Autodesk Inventor part; units mm, degrees
(part 3 of 3)
sketch "Sketch3" plane through (0, 0, 0) normal (0, -1, 0) x (1, 0, 0)
  circle A0 centre (-1.1015, 1.1015) radius 0.13 projected
  line L0 (-2.1254, 1.1532) -> (-2.1288, 1.1525) projected
  line L1 (-2.1288, 1.1525) -> (-2.1355, 1.1511) projected
  line L2 (-2.1355, 1.1511) -> (-2.149, 1.1477) projected
  line L3 (-2.149, 1.1477) -> (-2.1625, 1.1437) projected
  line L4 (-2.1625, 1.1437) -> (-2.1761, 1.139) projected
  line L5 (-2.1761, 1.139) -> (-2.1896, 1.1339) projected
  line L6 (-2.1896, 1.1339) -> (-2.2031, 1.1282) projected
  line L7 (-2.2031, 1.1282) -> (-2.2031, 1.0756) projected
  line L8 (-2.2031, 1.0756) -> (-2.1896, 1.0699) projected
  line L9 (-2.1896, 1.0699) -> (-2.1761, 1.0647) projected
  line L10 (-2.1761, 1.0647) -> (-2.1626, 1.0601) projected
  line L11 (-2.1626, 1.0601) -> (-2.1491, 1.0561) projected
  line L12 (-2.1491, 1.0561) -> (-2.1356, 1.0527) projected
  line L13 (-2.1356, 1.0527) -> (-2.1288, 1.0513) projected
  line L14 (-2.1288, 1.0513) -> (-2.1254, 1.0506) projected
  line L15 (-2.1254, 1.0506) -> (-2.1221, 1.05) projected
  line L16 (-2.1221, 1.05) -> (-2.1176, 0.9935) projected
  line L17 (-2.1176, 0.9935) -> (-2.1209, 0.9923) projected
  line L18 (-2.1209, 0.9923) -> (-2.1241, 0.9912) projected
  line L19 (-2.1241, 0.9912) -> (-2.1305, 0.9887) projected
  line L20 (-2.1305, 0.9887) -> (-2.1433, 0.9832) projected
  line L21 (-2.1433, 0.9832) -> (-2.156, 0.9772) projected
  line L22 (-2.156, 0.9772) -> (-2.1687, 0.9705) projected
  line L23 (-2.1687, 0.9705) -> (-2.1812, 0.9633) projected
  line L24 (-2.1812, 0.9633) -> (-2.1936, 0.9556) projected
  line L25 (-2.1936, 0.9556) -> (-2.1854, 0.9035) projected
  line L26 (-2.1854, 0.9035) -> (-2.1712, 0.9) projected
  line L27 (-2.1712, 0.9) -> (-2.1571, 0.897) projected
  line L28 (-2.1571, 0.897) -> (-2.143, 0.8945) projected
  line L29 (-2.143, 0.8945) -> (-2.129, 0.8927) projected
  line L30 (-2.129, 0.8927) -> (-2.1151, 0.8914) projected
  line L31 (-2.1151, 0.8914) -> (-2.1083, 0.8911) projected
  line L32 (-2.1083, 0.8911) -> (-2.1048, 0.891) projected
  line L33 (-2.1048, 0.891) -> (-2.1014, 0.8909) projected
  line L34 (-2.1014, 0.8909) -> (-2.0882, 0.8357) projected
  line L35 (-2.0882, 0.8357) -> (-2.0912, 0.8341) projected
  line L36 (-2.0912, 0.8341) -> (-2.0942, 0.8325) projected
  line L37 (-2.0942, 0.8325) -> (-2.1002, 0.829) projected
  line L38 (-2.1002, 0.829) -> (-2.112, 0.8216) projected
  line L39 (-2.112, 0.8216) -> (-2.1236, 0.8136) projected
  line L40 (-2.1236, 0.8136) -> (-2.135, 0.8051) projected
  line L41 (-2.135, 0.8051) -> (-2.1462, 0.796) projected
  line L42 (-2.1462, 0.796) -> (-2.1573, 0.7864) projected
  line L43 (-2.1573, 0.7864) -> (-2.1411, 0.7364) projected
  line L44 (-2.1411, 0.7364) -> (-2.1265, 0.7351) projected
  line L45 (-2.1265, 0.7351) -> (-2.112, 0.7344) projected
  line L46 (-2.112, 0.7344) -> (-2.0978, 0.7342) projected
  line L47 (-2.0978, 0.7342) -> (-2.0837, 0.7345) projected
  line L48 (-2.0837, 0.7345) -> (-2.0698, 0.7355) projected
  line L49 (-2.0698, 0.7355) -> (-2.0629, 0.7362) projected
  line L50 (-2.0629, 0.7362) -> (-2.0595, 0.7366) projected
  line L51 (-2.0595, 0.7366) -> (-2.0561, 0.7371) projected
  line L52 (-2.0561, 0.7371) -> (-2.0344, 0.6847) projected
  line L53 (-2.0344, 0.6847) -> (-2.0371, 0.6826) projected
  line L54 (-2.0371, 0.6826) -> (-2.0398, 0.6805) projected
  line L55 (-2.0398, 0.6805) -> (-2.0452, 0.6762) projected
  line L56 (-2.0452, 0.6762) -> (-2.0557, 0.667) projected
  line L57 (-2.0557, 0.667) -> (-2.0659, 0.6573) projected
  line L58 (-2.0659, 0.6573) -> (-2.0759, 0.6471) projected
  line L59 (-2.0759, 0.6471) -> (-2.0856, 0.6363) projected
  line L60 (-2.0856, 0.6363) -> (-2.095, 0.6252) projected
  line L61 (-2.095, 0.6252) -> (-2.0711, 0.5783) projected
  line L62 (-2.0711, 0.5783) -> (-2.0565, 0.5794) projected
  line L63 (-2.0565, 0.5794) -> (-2.0421, 0.5809) projected
  line L64 (-2.0421, 0.5809) -> (-2.028, 0.5829) projected
  line L65 (-2.028, 0.5829) -> (-2.0141, 0.5855) projected
  line L66 (-2.0141, 0.5855) -> (-2.0006, 0.5886) projected
  line L67 (-2.0006, 0.5886) -> (-1.9939, 0.5903) projected
  line L68 (-1.9939, 0.5903) -> (-1.9906, 0.5913) projected
  line L69 (-1.9906, 0.5913) -> (-1.9873, 0.5923) projected
  line L70 (-1.9873, 0.5923) -> (-1.9577, 0.5439) projected
  line L71 (-1.9577, 0.5439) -> (-1.9601, 0.5415) projected
  line L72 (-1.9601, 0.5415) -> (-1.9624, 0.5389) projected
  line L73 (-1.9624, 0.5389) -> (-1.967, 0.5338) projected
  line L74 (-1.967, 0.5338) -> (-1.976, 0.5231) projected
  line L75 (-1.976, 0.5231) -> (-1.9845, 0.5119) projected
  line L76 (-1.9845, 0.5119) -> (-1.9928, 0.5003) projected
  line L77 (-1.9928, 0.5003) -> (-2.0006, 0.4882) projected
  line L78 (-2.0006, 0.4882) -> (-2.0082, 0.4756) projected
  line L79 (-2.0082, 0.4756) -> (-1.9773, 0.4331) projected
  line L80 (-1.9773, 0.4331) -> (-1.9631, 0.4364) projected
  line L81 (-1.9631, 0.4364) -> (-1.9491, 0.4402) projected
  line L82 (-1.9491, 0.4402) -> (-1.9355, 0.4444) projected
  line L83 (-1.9355, 0.4444) -> (-1.9221, 0.4491) projected
  line L84 (-1.9221, 0.4491) -> (-1.9092, 0.4543) projected
  line L85 (-1.9092, 0.4543) -> (-1.9029, 0.4571) projected
  line L86 (-1.9029, 0.4571) -> (-1.8998, 0.4585) projected
  line L87 (-1.8998, 0.4585) -> (-1.8968, 0.46) projected
  line L88 (-1.8968, 0.46) -> (-1.8599, 0.4169) projected
  line L89 (-1.8599, 0.4169) -> (-1.8619, 0.4141) projected
  line L90 (-1.8619, 0.4141) -> (-1.8638, 0.4112) projected
  line L91 (-1.8638, 0.4112) -> (-1.8675, 0.4054) projected
  line L92 (-1.8675, 0.4054) -> (-1.8747, 0.3935) projected
  line L93 (-1.8747, 0.3935) -> (-1.8814, 0.3811) projected
  line L94 (-1.8814, 0.3811) -> (-1.8877, 0.3683) projected
  line L95 (-1.8877, 0.3683) -> (-1.8936, 0.3551) projected
  line L96 (-1.8936, 0.3551) -> (-1.8991, 0.3415) projected
  line L97 (-1.8991, 0.3415) -> (-1.8619, 0.3043) projected
  line L98 (-1.8619, 0.3043) -> (-1.8484, 0.3099) projected
  line L99 (-1.8484, 0.3099) -> (-1.8352, 0.3158) projected
  line L100 (-1.8352, 0.3158) -> (-1.8224, 0.3221) projected
  line L101 (-1.8224, 0.3221) -> (-1.81, 0.3288) projected
  line L102 (-1.81, 0.3288) -> (-1.798, 0.3359) projected
  line L103 (-1.798, 0.3359) -> (-1.7922, 0.3397) projected
  line L104 (-1.7922, 0.3397) -> (-1.7894, 0.3416) projected
  line L105 (-1.7894, 0.3416) -> (-1.7866, 0.3436) projected
  line L106 (-1.7866, 0.3436) -> (-1.7434, 0.3067) projected
  line L107 (-1.7434, 0.3067) -> (-1.7449, 0.3036) projected
  line L108 (-1.7449, 0.3036) -> (-1.7464, 0.3005) projected
  line L109 (-1.7464, 0.3005) -> (-1.7492, 0.2942) projected
  line L110 (-1.7492, 0.2942) -> (-1.7544, 0.2813) projected
  line L111 (-1.7544, 0.2813) -> (-1.7591, 0.268) projected
  line L112 (-1.7591, 0.268) -> (-1.7633, 0.2544) projected
  line L113 (-1.7633, 0.2544) -> (-1.7671, 0.2404) projected
  line L114 (-1.7671, 0.2404) -> (-1.7704, 0.2261) projected
  line L115 (-1.7704, 0.2261) -> (-1.7278, 0.1952) projected
  line L116 (-1.7278, 0.1952) -> (-1.7153, 0.2028) projected
  line L117 (-1.7153, 0.2028) -> (-1.7032, 0.2107) projected
  line L118 (-1.7032, 0.2107) -> (-1.6915, 0.2189) projected
  line L119 (-1.6915, 0.2189) -> (-1.6803, 0.2275) projected
  line L120 (-1.6803, 0.2275) -> (-1.6696, 0.2364) projected
  line L121 (-1.6696, 0.2364) -> (-1.6645, 0.241) projected
  line L122 (-1.6645, 0.241) -> (-1.662, 0.2434) projected
  line L123 (-1.662, 0.2434) -> (-1.6596, 0.2458) projected
  line L124 (-1.6596, 0.2458) -> (-1.6112, 0.2161) projected
  line L125 (-1.6112, 0.2161) -> (-1.6122, 0.2128) projected
  line L126 (-1.6122, 0.2128) -> (-1.6131, 0.2095) projected
  line L127 (-1.6131, 0.2095) -> (-1.6149, 0.2029) projected
  line L128 (-1.6149, 0.2029) -> (-1.618, 0.1893) projected
  line L129 (-1.618, 0.1893) -> (-1.6206, 0.1754) projected
  line L130 (-1.6206, 0.1754) -> (-1.6226, 0.1613) projected
  line L131 (-1.6226, 0.1613) -> (-1.6241, 0.1469) projected
  line L132 (-1.6241, 0.1469) -> (-1.6252, 0.1323) projected
  line L133 (-1.6252, 0.1323) -> (-1.5783, 0.1084) projected
  line L134 (-1.5783, 0.1084) -> (-1.5671, 0.1179) projected
  line L135 (-1.5671, 0.1179) -> (-1.5564, 0.1276) projected
  line L136 (-1.5564, 0.1276) -> (-1.5462, 0.1375) projected
  line L137 (-1.5462, 0.1375) -> (-1.5364, 0.1477) projected
  line L138 (-1.5364, 0.1477) -> (-1.5273, 0.1582) projected
  line L139 (-1.5273, 0.1582) -> (-1.5229, 0.1636) projected
  line L140 (-1.5229, 0.1636) -> (-1.5208, 0.1663) projected
  line L141 (-1.5208, 0.1663) -> (-1.5188, 0.169) projected
  line L142 (-1.5188, 0.169) -> (-1.4663, 0.1473) projected
  line L143 (-1.4663, 0.1473) -> (-1.4668, 0.1439) projected
  line L144 (-1.4668, 0.1439) -> (-1.4673, 0.1405) projected
  line L145 (-1.4673, 0.1405) -> (-1.468, 0.1337) projected
  line L146 (-1.468, 0.1337) -> (-1.4689, 0.1198) projected
  line L147 (-1.4689, 0.1198) -> (-1.4693, 0.1057) projected
  line L148 (-1.4693, 0.1057) -> (-1.469, 0.0914) projected
  line L149 (-1.469, 0.0914) -> (-1.4683, 0.077) projected
  line L150 (-1.4683, 0.077) -> (-1.4671, 0.0624) projected
  line L151 (-1.4671, 0.0624) -> (-1.4171, 0.0461) projected
  line L152 (-1.4171, 0.0461) -> (-1.4075, 0.0572) projected
  line L153 (-1.4075, 0.0572) -> (-1.3984, 0.0684) projected
  line L154 (-1.3984, 0.0684) -> (-1.3898, 0.0799) projected
  line L155 (-1.3898, 0.0799) -> (-1.3818, 0.0915) projected
  line L156 (-1.3818, 0.0915) -> (-1.3744, 0.1033) projected
  line L157 (-1.3744, 0.1033) -> (-1.371, 0.1092) projected
  line L158 (-1.371, 0.1092) -> (-1.3693, 0.1123) projected
  line L159 (-1.3693, 0.1123) -> (-1.3677, 0.1153) projected
  line L160 (-1.3677, 0.1153) -> (-1.3126, 0.102) projected
  line L161 (-1.3126, 0.102) -> (-1.3125, 0.0986) projected
  line L162 (-1.3125, 0.0986) -> (-1.3124, 0.0952) projected
  line L163 (-1.3124, 0.0952) -> (-1.312, 0.0883) projected
  line L164 (-1.312, 0.0883) -> (-1.3108, 0.0744) projected
  line L165 (-1.3108, 0.0744) -> (-1.3089, 0.0604) projected
  line L166 (-1.3089, 0.0604) -> (-1.3065, 0.0464) projected
  line L167 (-1.3065, 0.0464) -> (-1.3035, 0.0322) projected
  line L168 (-1.3035, 0.0322) -> (-1.3, 0.018) projected
  line L169 (-1.3, 0.018) -> (-1.248, 0.0098) projected
  line L170 (-1.248, 0.0098) -> (-1.2403, 0.0222) projected
  line L171 (-1.2403, 0.0222) -> (-1.2331, 0.0348) projected
  line L172 (-1.2331, 0.0348) -> (-1.2264, 0.0474) projected
  line L173 (-1.2264, 0.0474) -> (-1.2203, 0.0601) projected
  line L174 (-1.2203, 0.0601) -> (-1.2149, 0.0729) projected
  line L175 (-1.2149, 0.0729) -> (-1.2124, 0.0793) projected
  line L176 (-1.2124, 0.0793) -> (-1.2112, 0.0826) projected
  line L177 (-1.2112, 0.0826) -> (-1.2101, 0.0858) projected
  line L178 (-1.2101, 0.0858) -> (-1.1536, 0.0814) projected
  line L179 (-1.1536, 0.0814) -> (-1.153, 0.078) projected
  line L180 (-1.153, 0.078) -> (-1.1523, 0.0746) projected
  line L181 (-1.1523, 0.0746) -> (-1.1509, 0.0679) projected
  line L182 (-1.1509, 0.0679) -> (-1.1475, 0.0544) projected
  line L183 (-1.1475, 0.0544) -> (-1.1435, 0.0409) projected
  line L184 (-1.1435, 0.0409) -> (-1.1389, 0.0273) projected
  line L185 (-1.1389, 0.0273) -> (-1.1337, 0.0138) projected
  line L186 (-1.1337, 0.0138) -> (-1.128, 0.0003) projected
  line L187 (-1.128, 0.0003) -> (-1.0754, 0.0003) projected
  line L188 (-1.0754, 0.0003) -> (-1.0697, 0.0138) projected
  line L189 (-1.0697, 0.0138) -> (-1.0646, 0.0273) projected
  line L190 (-1.0646, 0.0273) -> (-1.06, 0.0409) projected
  line L191 (-1.06, 0.0409) -> (-1.0559, 0.0544) projected
  line L192 (-1.0559, 0.0544) -> (-1.0525, 0.0679) projected
  line L193 (-1.0525, 0.0679) -> (-1.0511, 0.0746) projected
  line L194 (-1.0511, 0.0746) -> (-1.0505, 0.078) projected
  line L195 (-1.0505, 0.078) -> (-1.0499, 0.0814) projected
  line L196 (-1.0499, 0.0814) -> (-0.9933, 0.0858) projected
  line L197 (-0.9933, 0.0858) -> (-0.9922, 0.0826) projected
  line L198 (-0.9922, 0.0826) -> (-0.991, 0.0793) projected
  line L199 (-0.991, 0.0793) -> (-0.9886, 0.0729) projected
  line L200 (-0.9886, 0.0729) -> (-0.9831, 0.0601) projected
  line L201 (-0.9831, 0.0601) -> (-0.977, 0.0474) projected
  line L202 (-0.977, 0.0474) -> (-0.9703, 0.0348) projected
  line L203 (-0.9703, 0.0348) -> (-0.9631, 0.0222) projected
  line L204 (-0.9631, 0.0222) -> (-0.9554, 0.0098) projected
  line L205 (-0.9554, 0.0098) -> (-0.9034, 0.018) projected
  line L206 (-0.9034, 0.018) -> (-0.9, 0.0322) projected
  line L207 (-0.9, 0.0322) -> (-0.897, 0.0464) projected
  line L208 (-0.897, 0.0464) -> (-0.8945, 0.0604) projected
  line L209 (-0.8945, 0.0604) -> (-0.8927, 0.0744) projected
  line L210 (-0.8927, 0.0744) -> (-0.8914, 0.0883) projected
  line L211 (-0.8914, 0.0883) -> (-0.8911, 0.0952) projected
  line L212 (-0.8911, 0.0952) -> (-0.891, 0.0986) projected
  line L213 (-0.891, 0.0986) -> (-0.8909, 0.102) projected
  line L214 (-0.8909, 0.102) -> (-0.8357, 0.1153) projected
  line L215 (-0.8357, 0.1153) -> (-0.8341, 0.1123) projected
  line L216 (-0.8341, 0.1123) -> (-0.8325, 0.1093) projected
  line L217 (-0.8325, 0.1093) -> (-0.829, 0.1033) projected
  line L218 (-0.829, 0.1033) -> (-0.8216, 0.0915) projected
  line L219 (-0.8216, 0.0915) -> (-0.8136, 0.0799) projected
  line L220 (-0.8136, 0.0799) -> (-0.805, 0.0685) projected
  line L221 (-0.805, 0.0685) -> (-0.796, 0.0572) projected
  line L222 (-0.796, 0.0572) -> (-0.7864, 0.0461) projected
  line L223 (-0.7864, 0.0461) -> (-0.7364, 0.0624) projected
  line L224 (-0.7364, 0.0624) -> (-0.7351, 0.077) projected
  line L225 (-0.7351, 0.077) -> (-0.7344, 0.0914) projected
  line L226 (-0.7344, 0.0914) -> (-0.7342, 0.1057) projected
  line L227 (-0.7342, 0.1057) -> (-0.7345, 0.1198) projected
  line L228 (-0.7345, 0.1198) -> (-0.7355, 0.1337) projected
  line L229 (-0.7355, 0.1337) -> (-0.7362, 0.1405) projected
  line L230 (-0.7362, 0.1405) -> (-0.7366, 0.1439) projected
  line L231 (-0.7366, 0.1439) -> (-0.7371, 0.1473) projected
  line L232 (-0.7371, 0.1473) -> (-0.6847, 0.169) projected
  line L233 (-0.6847, 0.169) -> (-0.6826, 0.1663) projected
  line L234 (-0.6826, 0.1663) -> (-0.6805, 0.1636) projected
  line L235 (-0.6805, 0.1636) -> (-0.6762, 0.1582) projected
  line L236 (-0.6762, 0.1582) -> (-0.667, 0.1477) projected
  line L237 (-0.667, 0.1477) -> (-0.6573, 0.1375) projected
  line L238 (-0.6573, 0.1375) -> (-0.647, 0.1276) projected
  line L239 (-0.647, 0.1276) -> (-0.6363, 0.1179) projected
  line L240 (-0.6363, 0.1179) -> (-0.6251, 0.1084) projected
  line L241 (-0.6251, 0.1084) -> (-0.5783, 0.1323) projected
  line L242 (-0.5783, 0.1323) -> (-0.5793, 0.1469) projected
  line L243 (-0.5793, 0.1469) -> (-0.5809, 0.1613) projected
  line L244 (-0.5809, 0.1613) -> (-0.5829, 0.1754) projected
  line L245 (-0.5829, 0.1754) -> (-0.5854, 0.1893) projected
  line L246 (-0.5854, 0.1893) -> (-0.5885, 0.2029) projected
  line L247 (-0.5885, 0.2029) -> (-0.5903, 0.2095) projected
  line L248 (-0.5903, 0.2095) -> (-0.5913, 0.2128) projected
  line L249 (-0.5913, 0.2128) -> (-0.5923, 0.2161) projected
  line L250 (-0.5923, 0.2161) -> (-0.5439, 0.2457) projected
  line L251 (-0.5439, 0.2457) -> (-0.5414, 0.2434) projected
  line L252 (-0.5414, 0.2434) -> (-0.5389, 0.241) projected
  line L253 (-0.5389, 0.241) -> (-0.5338, 0.2364) projected
  line L254 (-0.5338, 0.2364) -> (-0.5231, 0.2275) projected
  line L255 (-0.5231, 0.2275) -> (-0.5119, 0.2189) projected
  line L256 (-0.5119, 0.2189) -> (-0.5002, 0.2107) projected
  line L257 (-0.5002, 0.2107) -> (-0.4881, 0.2028) projected
  line L258 (-0.4881, 0.2028) -> (-0.4756, 0.1952) projected
  line L259 (-0.4756, 0.1952) -> (-0.4331, 0.2261) projected
  line L260 (-0.4331, 0.2261) -> (-0.4364, 0.2404) projected
  line L261 (-0.4364, 0.2404) -> (-0.4402, 0.2543) projected
  line L262 (-0.4402, 0.2543) -> (-0.4444, 0.268) projected
  line L263 (-0.4444, 0.268) -> (-0.449, 0.2813) projected
  line L264 (-0.449, 0.2813) -> (-0.4542, 0.2942) projected
  line L265 (-0.4542, 0.2942) -> (-0.457, 0.3005) projected
  line L266 (-0.457, 0.3005) -> (-0.4585, 0.3036) projected
  line L267 (-0.4585, 0.3036) -> (-0.46, 0.3067) projected
  line L268 (-0.46, 0.3067) -> (-0.4168, 0.3435) projected
  line L269 (-0.4168, 0.3435) -> (-0.414, 0.3416) projected
  line L270 (-0.414, 0.3416) -> (-0.4112, 0.3396) projected
  line L271 (-0.4112, 0.3396) -> (-0.4054, 0.3359) projected
  line L272 (-0.4054, 0.3359) -> (-0.3935, 0.3287) projected
  line L273 (-0.3935, 0.3287) -> (-0.3811, 0.322) projected
  line L274 (-0.3811, 0.322) -> (-0.3683, 0.3157) projected
  line L275 (-0.3683, 0.3157) -> (-0.3551, 0.3098) projected
  line L276 (-0.3551, 0.3098) -> (-0.3415, 0.3043) projected
  line L277 (-0.3415, 0.3043) -> (-0.3043, 0.3415) projected
  line L278 (-0.3043, 0.3415) -> (-0.3098, 0.3551) projected
  line L279 (-0.3098, 0.3551) -> (-0.3157, 0.3683) projected
  line L280 (-0.3157, 0.3683) -> (-0.322, 0.3811) projected
  line L281 (-0.322, 0.3811) -> (-0.3287, 0.3935) projected
  line L282 (-0.3287, 0.3935) -> (-0.3359, 0.4054) projected
  line L283 (-0.3359, 0.4054) -> (-0.3396, 0.4112) projected
  line L284 (-0.3396, 0.4112) -> (-0.3416, 0.4141) projected
  line L285 (-0.3416, 0.4141) -> (-0.3435, 0.4169) projected
  line L286 (-0.3435, 0.4169) -> (-0.3067, 0.46) projected
  line L287 (-0.3067, 0.46) -> (-0.3036, 0.4585) projected
  line L288 (-0.3036, 0.4585) -> (-0.3005, 0.457) projected
  line L289 (-0.3005, 0.457) -> (-0.2942, 0.4542) projected
  line L290 (-0.2942, 0.4542) -> (-0.2813, 0.449) projected
  line L291 (-0.2813, 0.449) -> (-0.268, 0.4444) projected
  line L292 (-0.268, 0.4444) -> (-0.2543, 0.4402) projected
  line L293 (-0.2543, 0.4402) -> (-0.2404, 0.4364) projected
  line L294 (-0.2404, 0.4364) -> (-0.2261, 0.4331) projected
  line L295 (-0.2261, 0.4331) -> (-0.1952, 0.4756) projected
  line L296 (-0.1952, 0.4756) -> (-0.2028, 0.4881) projected
  line L297 (-0.2028, 0.4881) -> (-0.2107, 0.5002) projected
  line L298 (-0.2107, 0.5002) -> (-0.2189, 0.5119) projected
  line L299 (-0.2189, 0.5119) -> (-0.2275, 0.5231) projected
  line L300 (-0.2275, 0.5231) -> (-0.2364, 0.5338) projected
  line L301 (-0.2364, 0.5338) -> (-0.241, 0.5389) projected
  line L302 (-0.241, 0.5389) -> (-0.2434, 0.5414) projected
  line L303 (-0.2434, 0.5414) -> (-0.2457, 0.5439) projected
  line L304 (-0.2457, 0.5439) -> (-0.2161, 0.5923) projected
  line L305 (-0.2161, 0.5923) -> (-0.2128, 0.5913) projected
  line L306 (-0.2128, 0.5913) -> (-0.2095, 0.5903) projected
  line L307 (-0.2095, 0.5903) -> (-0.2029, 0.5885) projected
  line L308 (-0.2029, 0.5885) -> (-0.1893, 0.5854) projected
  line L309 (-0.1893, 0.5854) -> (-0.1754, 0.5829) projected
  line L310 (-0.1754, 0.5829) -> (-0.1613, 0.5809) projected
  line L311 (-0.1613, 0.5809) -> (-0.1469, 0.5793) projected
  line L312 (-0.1469, 0.5793) -> (-0.1323, 0.5782) projected
  line L313 (-0.1323, 0.5782) -> (-0.1084, 0.6251) projected
  line L314 (-0.1084, 0.6251) -> (-0.1179, 0.6363) projected
  line L315 (-0.1179, 0.6363) -> (-0.1276, 0.647) projected
  line L316 (-0.1276, 0.647) -> (-0.1375, 0.6573) projected
  line L317 (-0.1375, 0.6573) -> (-0.1477, 0.667) projected
  line L318 (-0.1477, 0.667) -> (-0.1582, 0.6762) projected
  line L319 (-0.1582, 0.6762) -> (-0.1636, 0.6805) projected
  line L320 (-0.1636, 0.6805) -> (-0.1663, 0.6826) projected
  line L321 (-0.1663, 0.6826) -> (-0.169, 0.6847) projected
  line L322 (-0.169, 0.6847) -> (-0.1473, 0.7371) projected
  line L323 (-0.1473, 0.7371) -> (-0.1439, 0.7366) projected
  line L324 (-0.1439, 0.7366) -> (-0.1405, 0.7362) projected
  line L325 (-0.1405, 0.7362) -> (-0.1336, 0.7355) projected
  line L326 (-0.1336, 0.7355) -> (-0.1197, 0.7345) projected
  line L327 (-0.1197, 0.7345) -> (-0.1056, 0.7342) projected
  line L328 (-0.1056, 0.7342) -> (-0.0914, 0.7344) projected
  line L329 (-0.0914, 0.7344) -> (-0.0769, 0.7351) projected
  line L330 (-0.0769, 0.7351) -> (-0.0624, 0.7363) projected
  line L331 (-0.0624, 0.7363) -> (-0.0461, 0.7864) projected
  line L332 (-0.0461, 0.7864) -> (-0.0572, 0.7959) projected
  line L333 (-0.0572, 0.7959) -> (-0.0684, 0.805) projected
  line L334 (-0.0684, 0.805) -> (-0.0799, 0.8136) projected
  line L335 (-0.0799, 0.8136) -> (-0.0915, 0.8216) projected
  line L336 (-0.0915, 0.8216) -> (-0.1033, 0.829) projected
  line L337 (-0.1033, 0.829) -> (-0.1092, 0.8324) projected
  line L338 (-0.1092, 0.8324) -> (-0.1122, 0.8341) projected
  line L339 (-0.1122, 0.8341) -> (-0.1153, 0.8357) projected
  line L340 (-0.1153, 0.8357) -> (-0.102, 0.8909) projected
  line L341 (-0.102, 0.8909) -> (-0.0986, 0.8909) projected
  line L342 (-0.0986, 0.8909) -> (-0.0952, 0.891) projected
  line L343 (-0.0952, 0.891) -> (-0.0883, 0.8914) projected
  line L344 (-0.0883, 0.8914) -> (-0.0744, 0.8926) projected
  line L345 (-0.0744, 0.8926) -> (-0.0604, 0.8945) projected
  line L346 (-0.0604, 0.8945) -> (-0.0464, 0.897) projected
  line L347 (-0.0464, 0.897) -> (-0.0322, 0.8999) projected
  line L348 (-0.0322, 0.8999) -> (-0.018, 0.9034) projected
  line L349 (-0.018, 0.9034) -> (-0.0098, 0.9554) projected
  line L350 (-0.0098, 0.9554) -> (-0.0222, 0.9631) projected
  line L351 (-0.0222, 0.9631) -> (-0.0347, 0.9703) projected
  line L352 (-0.0347, 0.9703) -> (-0.0474, 0.977) projected
  line L353 (-0.0474, 0.977) -> (-0.0601, 0.9831) projected
  line L354 (-0.0601, 0.9831) -> (-0.0729, 0.9885) projected
  line L355 (-0.0729, 0.9885) -> (-0.0793, 0.991) projected
  line L356 (-0.0793, 0.991) -> (-0.0825, 0.9922) projected
  line L357 (-0.0825, 0.9922) -> (-0.0858, 0.9933) projected
  line L358 (-0.0858, 0.9933) -> (-0.0813, 1.0499) projected
  line L359 (-0.0813, 1.0499) -> (-0.078, 1.0505) projected
  line L360 (-0.078, 1.0505) -> (-0.0746, 1.0511) projected
  line L361 (-0.0746, 1.0511) -> (-0.0678, 1.0525) projected
  line L362 (-0.0678, 1.0525) -> (-0.0543, 1.0559) projected
  line L363 (-0.0543, 1.0559) -> (-0.0408, 1.06) projected
  line L364 (-0.0408, 1.06) -> (-0.0273, 1.0646) projected
  line L365 (-0.0273, 1.0646) -> (-0.0138, 1.0697) projected
  line L366 (-0.0138, 1.0697) -> (-0.0003, 1.0754) projected
  line L367 (-0.0003, 1.0754) -> (-0.0003, 1.128) projected
  line L368 (-0.0003, 1.128) -> (-0.0138, 1.1337) projected
  line L369 (-0.0138, 1.1337) -> (-0.0273, 1.1388) projected
  line L370 (-0.0273, 1.1388) -> (-0.0408, 1.1435) projected
  line L371 (-0.0408, 1.1435) -> (-0.0543, 1.1475) projected
  line L372 (-0.0543, 1.1475) -> (-0.0678, 1.1509) projected
  line L373 (-0.0678, 1.1509) -> (-0.0746, 1.1523) projected
  line L374 (-0.0746, 1.1523) -> (-0.078, 1.153) projected
  line L375 (-0.078, 1.153) -> (-0.0813, 1.1536) projected
  line L376 (-0.0813, 1.1536) -> (-0.0858, 1.2101) projected
  line L377 (-0.0858, 1.2101) -> (-0.0825, 1.2112) projected
  line L378 (-0.0825, 1.2112) -> (-0.0793, 1.2124) projected
  line L379 (-0.0793, 1.2124) -> (-0.0729, 1.2149) projected
  line L380 (-0.0729, 1.2149) -> (-0.0601, 1.2203) projected
  line L381 (-0.0601, 1.2203) -> (-0.0474, 1.2264) projected
  line L382 (-0.0474, 1.2264) -> (-0.0347, 1.2331) projected
  line L383 (-0.0347, 1.2331) -> (-0.0222, 1.2403) projected
  line L384 (-0.0222, 1.2403) -> (-0.0098, 1.248) projected
  line L385 (-0.0098, 1.248) -> (-0.018, 1.3) projected
  line L386 (-0.018, 1.3) -> (-0.0322, 1.3035) projected
  line L387 (-0.0322, 1.3035) -> (-0.0464, 1.3065) projected
  line L388 (-0.0464, 1.3065) -> (-0.0604, 1.3089) projected
  line L389 (-0.0604, 1.3089) -> (-0.0744, 1.3108) projected
  line L390 (-0.0744, 1.3108) -> (-0.0883, 1.312) projected
  line L391 (-0.0883, 1.312) -> (-0.0952, 1.3124) projected
  line L392 (-0.0952, 1.3124) -> (-0.0986, 1.3125) projected
  line L393 (-0.0986, 1.3125) -> (-0.102, 1.3125) projected
  line L394 (-0.102, 1.3125) -> (-0.1153, 1.3677) projected
  line L395 (-0.1153, 1.3677) -> (-0.1122, 1.3693) projected
  line L396 (-0.1122, 1.3693) -> (-0.1092, 1.371) projected
  line L397 (-0.1092, 1.371) -> (-0.1033, 1.3744) projected
  line L398 (-0.1033, 1.3744) -> (-0.0915, 1.3818) projected
  line L399 (-0.0915, 1.3818) -> (-0.0799, 1.3898) projected
  line L400 (-0.0799, 1.3898) -> (-0.0684, 1.3984) projected
  line L401 (-0.0684, 1.3984) -> (-0.0572, 1.4075) projected
  line L402 (-0.0572, 1.4075) -> (-0.0461, 1.417) projected
  line L403 (-0.0461, 1.417) -> (-0.0624, 1.4671) projected
  line L404 (-0.0624, 1.4671) -> (-0.0769, 1.4683) projected
  line L405 (-0.0769, 1.4683) -> (-0.0914, 1.469) projected
  line L406 (-0.0914, 1.469) -> (-0.1056, 1.4692) projected
  line L407 (-0.1056, 1.4692) -> (-0.1197, 1.4689) projected
  line L408 (-0.1197, 1.4689) -> (-0.1336, 1.468) projected
  line L409 (-0.1336, 1.468) -> (-0.1405, 1.4672) projected
  line L410 (-0.1405, 1.4672) -> (-0.1439, 1.4668) projected
  line L411 (-0.1439, 1.4668) -> (-0.1473, 1.4663) projected
  line L412 (-0.1473, 1.4663) -> (-0.169, 1.5188) projected
  line L413 (-0.169, 1.5188) -> (-0.1663, 1.5208) projected
  line L414 (-0.1663, 1.5208) -> (-0.1636, 1.5229) projected
  line L415 (-0.1636, 1.5229) -> (-0.1582, 1.5273) projected
  line L416 (-0.1582, 1.5273) -> (-0.1477, 1.5364) projected
  line L417 (-0.1477, 1.5364) -> (-0.1375, 1.5461) projected
  line L418 (-0.1375, 1.5461) -> (-0.1275, 1.5564) projected
  line L419 (-0.1275, 1.5564) -> (-0.1179, 1.5671) projected
  line L420 (-0.1179, 1.5671) -> (-0.1084, 1.5783) projected
  line L421 (-0.1084, 1.5783) -> (-0.1323, 1.6252) projected
  line L422 (-0.1323, 1.6252) -> (-0.1469, 1.6241) projected
  line L423 (-0.1469, 1.6241) -> (-0.1613, 1.6226) projected
  line L424 (-0.1613, 1.6226) -> (-0.1754, 1.6205) projected
  line L425 (-0.1754, 1.6205) -> (-0.1893, 1.618) projected
  line L426 (-0.1893, 1.618) -> (-0.2028, 1.6149) projected
  line L427 (-0.2028, 1.6149) -> (-0.2095, 1.6131) projected
  line L428 (-0.2095, 1.6131) -> (-0.2128, 1.6122) projected
  line L429 (-0.2128, 1.6122) -> (-0.2161, 1.6112) projected
  line L430 (-0.2161, 1.6112) -> (-0.2457, 1.6595) projected
  line L431 (-0.2457, 1.6595) -> (-0.2433, 1.662) projected
  line L432 (-0.2433, 1.662) -> (-0.241, 1.6645) projected
  line L433 (-0.241, 1.6645) -> (-0.2364, 1.6696) projected
  line L434 (-0.2364, 1.6696) -> (-0.2274, 1.6803) projected
  line L435 (-0.2274, 1.6803) -> (-0.2189, 1.6915) projected
  line L436 (-0.2189, 1.6915) -> (-0.2106, 1.7032) projected
  line L437 (-0.2106, 1.7032) -> (-0.2028, 1.7153) projected
  line L438 (-0.2028, 1.7153) -> (-0.1952, 1.7278) projected
  line L439 (-0.1952, 1.7278) -> (-0.2261, 1.7704) projected
  line L440 (-0.2261, 1.7704) -> (-0.2403, 1.767) projected
  line L441 (-0.2403, 1.767) -> (-0.2543, 1.7633) projected
  line L442 (-0.2543, 1.7633) -> (-0.268, 1.7591) projected
  line L443 (-0.268, 1.7591) -> (-0.2813, 1.7544) projected
  line L444 (-0.2813, 1.7544) -> (-0.2942, 1.7492) projected
  line L445 (-0.2942, 1.7492) -> (-0.3005, 1.7464) projected
  line L446 (-0.3005, 1.7464) -> (-0.3036, 1.7449) projected
  line L447 (-0.3036, 1.7449) -> (-0.3067, 1.7434) projected
  line L448 (-0.3067, 1.7434) -> (-0.3435, 1.7866) projected
  line L449 (-0.3435, 1.7866) -> (-0.3415, 1.7894) projected
  line L450 (-0.3415, 1.7894) -> (-0.3396, 1.7922) projected
  line L451 (-0.3396, 1.7922) -> (-0.3358, 1.798) projected
  line L452 (-0.3358, 1.798) -> (-0.3287, 1.8099) projected
  line L453 (-0.3287, 1.8099) -> (-0.322, 1.8224) projected
  line L454 (-0.322, 1.8224) -> (-0.3157, 1.8352) projected
  line L455 (-0.3157, 1.8352) -> (-0.3098, 1.8484) projected
  line L456 (-0.3098, 1.8484) -> (-0.3043, 1.8619) projected
  line L457 (-0.3043, 1.8619) -> (-0.3415, 1.8991) projected
  line L458 (-0.3415, 1.8991) -> (-0.355, 1.8936) projected
  line L459 (-0.355, 1.8936) -> (-0.3682, 1.8877) projected
  line L460 (-0.3682, 1.8877) -> (-0.381, 1.8814) projected
  line L461 (-0.381, 1.8814) -> (-0.3934, 1.8747) projected
  line L462 (-0.3934, 1.8747) -> (-0.4054, 1.8676) projected
  line L463 (-0.4054, 1.8676) -> (-0.4112, 1.8638) projected
  line L464 (-0.4112, 1.8638) -> (-0.414, 1.8619) projected
  line L465 (-0.414, 1.8619) -> (-0.4168, 1.8599) projected
  line L466 (-0.4168, 1.8599) -> (-0.46, 1.8968) projected
  line L467 (-0.46, 1.8968) -> (-0.4585, 1.8998) projected
  line L468 (-0.4585, 1.8998) -> (-0.457, 1.9029) projected
  line L469 (-0.457, 1.9029) -> (-0.4542, 1.9092) projected
  line L470 (-0.4542, 1.9092) -> (-0.449, 1.9222) projected
  line L471 (-0.449, 1.9222) -> (-0.4443, 1.9355) projected
  line L472 (-0.4443, 1.9355) -> (-0.4401, 1.9491) projected
  line L473 (-0.4401, 1.9491) -> (-0.4363, 1.9631) projected
  line L474 (-0.4363, 1.9631) -> (-0.433, 1.9773) projected
  line L475 (-0.433, 1.9773) -> (-0.4756, 2.0082) projected
  line L476 (-0.4756, 2.0082) -> (-0.4881, 2.0007) projected
  line L477 (-0.4881, 2.0007) -> (-0.5002, 1.9928) projected
  line L478 (-0.5002, 1.9928) -> (-0.5119, 1.9845) projected
  line L479 (-0.5119, 1.9845) -> (-0.5231, 1.976) projected
  line L480 (-0.5231, 1.976) -> (-0.5338, 1.967) projected
  line L481 (-0.5338, 1.967) -> (-0.5389, 1.9624) projected
  line L482 (-0.5389, 1.9624) -> (-0.5414, 1.9601) projected
  line L483 (-0.5414, 1.9601) -> (-0.5438, 1.9577) projected
  line L484 (-0.5438, 1.9577) -> (-0.5922, 1.9874) projected
  line L485 (-0.5922, 1.9874) -> (-0.5912, 1.9906) projected
  line L486 (-0.5912, 1.9906) -> (-0.5903, 1.9939) projected
  line L487 (-0.5903, 1.9939) -> (-0.5885, 2.0006) projected
  line L488 (-0.5885, 2.0006) -> (-0.5854, 2.0142) projected
  line L489 (-0.5854, 2.0142) -> (-0.5828, 2.028) projected
  line L490 (-0.5828, 2.028) -> (-0.5808, 2.0422) projected
  line L491 (-0.5808, 2.0422) -> (-0.5793, 2.0565) projected
  line L492 (-0.5793, 2.0565) -> (-0.5782, 2.0711) projected
  line L493 (-0.5782, 2.0711) -> (-0.6251, 2.095) projected
  line L494 (-0.6251, 2.095) -> (-0.6363, 2.0856) projected
  line L495 (-0.6363, 2.0856) -> (-0.647, 2.0759) projected
  line L496 (-0.647, 2.0759) -> (-0.6572, 2.0659) projected
  line L497 (-0.6572, 2.0659) -> (-0.667, 2.0557) projected
  line L498 (-0.667, 2.0557) -> (-0.6761, 2.0452) projected
  line L499 (-0.6761, 2.0452) -> (-0.6805, 2.0399) projected
  line L500 (-0.6805, 2.0399) -> (-0.6826, 2.0372) projected
  line L501 (-0.6826, 2.0372) -> (-0.6846, 2.0344) projected
  line L502 (-0.6846, 2.0344) -> (-0.737, 2.0562) projected
  line L503 (-0.737, 2.0562) -> (-0.7366, 2.0595) projected
  line L504 (-0.7366, 2.0595) -> (-0.7361, 2.0629) projected
  line L505 (-0.7361, 2.0629) -> (-0.7354, 2.0698) projected
  line L506 (-0.7354, 2.0698) -> (-0.7345, 2.0837) projected
  line L507 (-0.7345, 2.0837) -> (-0.7341, 2.0978) projected
  line L508 (-0.7341, 2.0978) -> (-0.7343, 2.1121) projected
  line L509 (-0.7343, 2.1121) -> (-0.7351, 2.1265) projected
  line L510 (-0.7351, 2.1265) -> (-0.7363, 2.1411) projected
  line L511 (-0.7363, 2.1411) -> (-0.7863, 2.1573) projected
  line L512 (-0.7863, 2.1573) -> (-0.7959, 2.1463) projected
  line L513 (-0.7959, 2.1463) -> (-0.805, 2.135) projected
  line L514 (-0.805, 2.135) -> (-0.8135, 2.1236) projected
  line L515 (-0.8135, 2.1236) -> (-0.8215, 2.112) projected
  line L516 (-0.8215, 2.112) -> (-0.8289, 2.1002) projected
  line L517 (-0.8289, 2.1002) -> (-0.8324, 2.0942) projected
  line L518 (-0.8324, 2.0942) -> (-0.8341, 2.0912) projected
  line L519 (-0.8341, 2.0912) -> (-0.8357, 2.0882) projected
  line L520 (-0.8357, 2.0882) -> (-0.8908, 2.1014) projected
  line L521 (-0.8908, 2.1014) -> (-0.8909, 2.1049) projected
  line L522 (-0.8909, 2.1049) -> (-0.891, 2.1083) projected
  line L523 (-0.891, 2.1083) -> (-0.8914, 2.1152) projected
  line L524 (-0.8914, 2.1152) -> (-0.8926, 2.129) projected
  line L525 (-0.8926, 2.129) -> (-0.8945, 2.143) projected
  line L526 (-0.8945, 2.143) -> (-0.8969, 2.1571) projected
  line L527 (-0.8969, 2.1571) -> (-0.8999, 2.1712) projected
  line L528 (-0.8999, 2.1712) -> (-0.9034, 2.1855) projected
  line L529 (-0.9034, 2.1855) -> (-0.9553, 2.1937) projected
  line L530 (-0.9553, 2.1937) -> (-0.9631, 2.1812) projected
  line L531 (-0.9631, 2.1812) -> (-0.9703, 2.1687) projected
  line L532 (-0.9703, 2.1687) -> (-0.9769, 2.1561) projected
  line L533 (-0.9769, 2.1561) -> (-0.983, 2.1434) projected
  line L534 (-0.983, 2.1434) -> (-0.9885, 2.1306) projected
  line L535 (-0.9885, 2.1306) -> (-0.991, 2.1241) projected
  line L536 (-0.991, 2.1241) -> (-0.9921, 2.1209) projected
  line L537 (-0.9921, 2.1209) -> (-0.9932, 2.1177) projected
  line L538 (-0.9932, 2.1177) -> (-1.0498, 2.1221) projected
  line L539 (-1.0498, 2.1221) -> (-1.0504, 2.1255) projected
  line L540 (-1.0504, 2.1255) -> (-1.0511, 2.1289) projected
  line L541 (-1.0511, 2.1289) -> (-1.0525, 2.1356) projected
  line L542 (-1.0525, 2.1356) -> (-1.0559, 2.1491) projected
  line L543 (-1.0559, 2.1491) -> (-1.0599, 2.1626) projected
  line L544 (-1.0599, 2.1626) -> (-1.0645, 2.1761) projected
  line L545 (-1.0645, 2.1761) -> (-1.0697, 2.1896) projected
  line L546 (-1.0697, 2.1896) -> (-1.0754, 2.2031) projected
  line L547 (-1.0754, 2.2031) -> (-1.128, 2.2031) projected
  line L548 (-1.128, 2.2031) -> (-1.1336, 2.1896) projected
  line L549 (-1.1336, 2.1896) -> (-1.1388, 2.1761) projected
  line L550 (-1.1388, 2.1761) -> (-1.1434, 2.1626) projected
  line L551 (-1.1434, 2.1626) -> (-1.1474, 2.1491) projected
  line L552 (-1.1474, 2.1491) -> (-1.1508, 2.1356) projected
  line L553 (-1.1508, 2.1356) -> (-1.1523, 2.1289) projected
  line L554 (-1.1523, 2.1289) -> (-1.1529, 2.1255) projected
  line L555 (-1.1529, 2.1255) -> (-1.1535, 2.1221) projected
  line L556 (-1.1535, 2.1221) -> (-1.2101, 2.1177) projected
  line L557 (-1.2101, 2.1177) -> (-1.2112, 2.1209) projected
  line L558 (-1.2112, 2.1209) -> (-1.2124, 2.1241) projected
  line L559 (-1.2124, 2.1241) -> (-1.2148, 2.1306) projected
  line L560 (-1.2148, 2.1306) -> (-1.2203, 2.1434) projected
  line L561 (-1.2203, 2.1434) -> (-1.2264, 2.1561) projected
  line L562 (-1.2264, 2.1561) -> (-1.2331, 2.1687) projected
  line L563 (-1.2331, 2.1687) -> (-1.2403, 2.1812) projected
  line L564 (-1.2403, 2.1812) -> (-1.248, 2.1937) projected
  line L565 (-1.248, 2.1937) -> (-1.2999, 2.1855) projected
  line L566 (-1.2999, 2.1855) -> (-1.3034, 2.1712) projected
  line L567 (-1.3034, 2.1712) -> (-1.3064, 2.1571) projected
  line L568 (-1.3064, 2.1571) -> (-1.3089, 2.143) projected
  line L569 (-1.3089, 2.143) -> (-1.3107, 2.129) projected
  line L570 (-1.3107, 2.129) -> (-1.312, 2.1152) projected
  line L571 (-1.312, 2.1152) -> (-1.3123, 2.1083) projected
  line L572 (-1.3123, 2.1083) -> (-1.3124, 2.1049) projected
  line L573 (-1.3124, 2.1049) -> (-1.3125, 2.1014) projected
  line L574 (-1.3125, 2.1014) -> (-1.3677, 2.0882) projected
  line L575 (-1.3677, 2.0882) -> (-1.3693, 2.0912) projected
  line L576 (-1.3693, 2.0912) -> (-1.3709, 2.0942) projected
  line L577 (-1.3709, 2.0942) -> (-1.3744, 2.1002) projected
  line L578 (-1.3744, 2.1002) -> (-1.3818, 2.112) projected
  line L579 (-1.3818, 2.112) -> (-1.3898, 2.1236) projected
  line L580 (-1.3898, 2.1236) -> (-1.3983, 2.135) projected
  line L581 (-1.3983, 2.135) -> (-1.4074, 2.1463) projected
  line L582 (-1.4074, 2.1463) -> (-1.417, 2.1573) projected
  line L583 (-1.417, 2.1573) -> (-1.467, 2.1411) projected
  line L584 (-1.467, 2.1411) -> (-1.4683, 2.1265) projected
  line L585 (-1.4683, 2.1265) -> (-1.469, 2.1121) projected
  line L586 (-1.469, 2.1121) -> (-1.4692, 2.0978) projected
  line L587 (-1.4692, 2.0978) -> (-1.4689, 2.0837) projected
  line L588 (-1.4689, 2.0837) -> (-1.4679, 2.0698) projected
  line L589 (-1.4679, 2.0698) -> (-1.4672, 2.0629) projected
  line L590 (-1.4672, 2.0629) -> (-1.4668, 2.0595) projected
  line L591 (-1.4668, 2.0595) -> (-1.4663, 2.0562) projected
  line L592 (-1.4663, 2.0562) -> (-1.5187, 2.0344) projected
  line L593 (-1.5187, 2.0344) -> (-1.5208, 2.0372) projected
  line L594 (-1.5208, 2.0372) -> (-1.5229, 2.0399) projected
  line L595 (-1.5229, 2.0399) -> (-1.5272, 2.0452) projected
  line L596 (-1.5272, 2.0452) -> (-1.5364, 2.0557) projected
  line L597 (-1.5364, 2.0557) -> (-1.5461, 2.0659) projected
  line L598 (-1.5461, 2.0659) -> (-1.5563, 2.0759) projected
  line L599 (-1.5563, 2.0759) -> (-1.5671, 2.0856) projected
  line L600 (-1.5671, 2.0856) -> (-1.5783, 2.095) projected
  line L601 (-1.5783, 2.095) -> (-1.6251, 2.0711) projected
  line L602 (-1.6251, 2.0711) -> (-1.6241, 2.0566) projected
  line L603 (-1.6241, 2.0566) -> (-1.6225, 2.0422) projected
  line L604 (-1.6225, 2.0422) -> (-1.6205, 2.028) projected
  line L605 (-1.6205, 2.028) -> (-1.6179, 2.0142) projected
  line L606 (-1.6179, 2.0142) -> (-1.6149, 2.0006) projected
  line L607 (-1.6149, 2.0006) -> (-1.6131, 1.9939) projected
  line L608 (-1.6131, 1.9939) -> (-1.6121, 1.9906) projected
  line L609 (-1.6121, 1.9906) -> (-1.6111, 1.9874) projected
  line L610 (-1.6111, 1.9874) -> (-1.6595, 1.9577) projected
  line L611 (-1.6595, 1.9577) -> (-1.662, 1.9601) projected
  line L612 (-1.662, 1.9601) -> (-1.6645, 1.9624) projected
  line L613 (-1.6645, 1.9624) -> (-1.6696, 1.9671) projected
  line L614 (-1.6696, 1.9671) -> (-1.6803, 1.976) projected
  line L615 (-1.6803, 1.976) -> (-1.6915, 1.9846) projected
  line L616 (-1.6915, 1.9846) -> (-1.7031, 1.9928) projected
  line L617 (-1.7031, 1.9928) -> (-1.7153, 2.0007) projected
  line L618 (-1.7153, 2.0007) -> (-1.7278, 2.0083) projected
  line L619 (-1.7278, 2.0083) -> (-1.7703, 1.9773) projected
  line L620 (-1.7703, 1.9773) -> (-1.767, 1.9631) projected
  line L621 (-1.767, 1.9631) -> (-1.7632, 1.9491) projected
  line L622 (-1.7632, 1.9491) -> (-1.759, 1.9355) projected
  line L623 (-1.759, 1.9355) -> (-1.7543, 1.9222) projected
  line L624 (-1.7543, 1.9222) -> (-1.7491, 1.9093) projected
  line L625 (-1.7491, 1.9093) -> (-1.7463, 1.903) projected
  line L626 (-1.7463, 1.903) -> (-1.7449, 1.8999) projected
  line L627 (-1.7449, 1.8999) -> (-1.7434, 1.8968) projected
  line L628 (-1.7434, 1.8968) -> (-1.7865, 1.8599) projected
  line L629 (-1.7865, 1.8599) -> (-1.7893, 1.8619) projected
  line L630 (-1.7893, 1.8619) -> (-1.7922, 1.8638) projected
  line L631 (-1.7922, 1.8638) -> (-1.798, 1.8676) projected
  line L632 (-1.798, 1.8676) -> (-1.8099, 1.8747) projected
  line L633 (-1.8099, 1.8747) -> (-1.8223, 1.8814) projected
  line L634 (-1.8223, 1.8814) -> (-1.8351, 1.8877) projected
  line L635 (-1.8351, 1.8877) -> (-1.8483, 1.8936) projected
  line L636 (-1.8483, 1.8936) -> (-1.8619, 1.8992) projected
  line L637 (-1.8619, 1.8992) -> (-1.8991, 1.862) projected
  line L638 (-1.8991, 1.862) -> (-1.8936, 1.8484) projected
  line L639 (-1.8936, 1.8484) -> (-1.8877, 1.8352) projected
  line L640 (-1.8877, 1.8352) -> (-1.8814, 1.8224) projected
  line L641 (-1.8814, 1.8224) -> (-1.8747, 1.81) projected
  line L642 (-1.8747, 1.81) -> (-1.8675, 1.798) projected
  line L643 (-1.8675, 1.798) -> (-1.8637, 1.7923) projected
  line L644 (-1.8637, 1.7923) -> (-1.8618, 1.7894) projected
  line L645 (-1.8618, 1.7894) -> (-1.8599, 1.7866) projected
  line L646 (-1.8599, 1.7866) -> (-1.8967, 1.7435) projected
  line L647 (-1.8967, 1.7435) -> (-1.8998, 1.745) projected
  line L648 (-1.8998, 1.745) -> (-1.9029, 1.7464) projected
  line L649 (-1.9029, 1.7464) -> (-1.9092, 1.7492) projected
  line L650 (-1.9092, 1.7492) -> (-1.9221, 1.7544) projected
  line L651 (-1.9221, 1.7544) -> (-1.9354, 1.7591) projected
  line L652 (-1.9354, 1.7591) -> (-1.9491, 1.7633) projected
  line L653 (-1.9491, 1.7633) -> (-1.963, 1.7671) projected
  line L654 (-1.963, 1.7671) -> (-1.9773, 1.7704) projected
  line L655 (-1.9773, 1.7704) -> (-2.0082, 1.7279) projected
  line L656 (-2.0082, 1.7279) -> (-2.0006, 1.7153) projected
  line L657 (-2.0006, 1.7153) -> (-1.9927, 1.7032) projected
  line L658 (-1.9927, 1.7032) -> (-1.9845, 1.6916) projected
  line L659 (-1.9845, 1.6916) -> (-1.9759, 1.6804) projected
  line L660 (-1.9759, 1.6804) -> (-1.967, 1.6697) projected
  line L661 (-1.967, 1.6697) -> (-1.9624, 1.6645) projected
  line L662 (-1.9624, 1.6645) -> (-1.96, 1.662) projected
  line L663 (-1.96, 1.662) -> (-1.9577, 1.6596) projected
  line L664 (-1.9577, 1.6596) -> (-1.9873, 1.6112) projected
  line L665 (-1.9873, 1.6112) -> (-1.9906, 1.6122) projected
  line L666 (-1.9906, 1.6122) -> (-1.9939, 1.6132) projected
  line L667 (-1.9939, 1.6132) -> (-2.0005, 1.6149) projected
  line L668 (-2.0005, 1.6149) -> (-2.0141, 1.618) projected
  line L669 (-2.0141, 1.618) -> (-2.028, 1.6206) projected
  line L670 (-2.028, 1.6206) -> (-2.0421, 1.6226) projected
  line L671 (-2.0421, 1.6226) -> (-2.0565, 1.6242) projected
  line L672 (-2.0565, 1.6242) -> (-2.0711, 1.6252) projected
  line L673 (-2.0711, 1.6252) -> (-2.095, 1.5783) projected
  line L674 (-2.095, 1.5783) -> (-2.0855, 1.5672) projected
  line L675 (-2.0855, 1.5672) -> (-2.0758, 1.5564) projected
  line L676 (-2.0758, 1.5564) -> (-2.0659, 1.5462) projected
  line L677 (-2.0659, 1.5462) -> (-2.0557, 1.5365) projected
  line L678 (-2.0557, 1.5365) -> (-2.0452, 1.5273) projected
  line L679 (-2.0452, 1.5273) -> (-2.0398, 1.523) projected
  line L680 (-2.0398, 1.523) -> (-2.0371, 1.5209) projected
  line L681 (-2.0371, 1.5209) -> (-2.0344, 1.5188) projected
  line L682 (-2.0344, 1.5188) -> (-2.0561, 1.4664) projected
  line L683 (-2.0561, 1.4664) -> (-2.0595, 1.4669) projected
  line L684 (-2.0595, 1.4669) -> (-2.0629, 1.4673) projected
  line L685 (-2.0629, 1.4673) -> (-2.0697, 1.468) projected
  line L686 (-2.0697, 1.468) -> (-2.0836, 1.469) projected
  line L687 (-2.0836, 1.469) -> (-2.0977, 1.4693) projected
  line L688 (-2.0977, 1.4693) -> (-2.112, 1.4691) projected
  line L689 (-2.112, 1.4691) -> (-2.1265, 1.4684) projected
  line L690 (-2.1265, 1.4684) -> (-2.141, 1.4671) projected
  line L691 (-2.141, 1.4671) -> (-2.1573, 1.4171) projected
  line L692 (-2.1573, 1.4171) -> (-2.1462, 1.4075) projected
  line L693 (-2.1462, 1.4075) -> (-2.135, 1.3984) projected
  line L694 (-2.135, 1.3984) -> (-2.1235, 1.3899) projected
  line L695 (-2.1235, 1.3899) -> (-2.1119, 1.3819) projected
  line L696 (-2.1119, 1.3819) -> (-2.1001, 1.3745) projected
  line L697 (-2.1001, 1.3745) -> (-2.0942, 1.371) projected
  line L698 (-2.0942, 1.371) -> (-2.0912, 1.3694) projected
  line L699 (-2.0912, 1.3694) -> (-2.0881, 1.3678) projected
  line L700 (-2.0881, 1.3678) -> (-2.1014, 1.3126) projected
  line L701 (-2.1014, 1.3126) -> (-2.1048, 1.3125) projected
  line L702 (-2.1048, 1.3125) -> (-2.1082, 1.3124) projected
  line L703 (-2.1082, 1.3124) -> (-2.1151, 1.3121) projected
  line L704 (-2.1151, 1.3121) -> (-2.129, 1.3108) projected
  line L705 (-2.129, 1.3108) -> (-2.143, 1.3089) projected
  line L706 (-2.143, 1.3089) -> (-2.157, 1.3065) projected
  line L707 (-2.157, 1.3065) -> (-2.1712, 1.3035) projected
  line L708 (-2.1712, 1.3035) -> (-2.1854, 1.3) projected
  line L709 (-2.1854, 1.3) -> (-2.1936, 1.2482) projected
  line L710 (-2.1936, 1.2482) -> (-2.1812, 1.2405) projected
  line L711 (-2.1812, 1.2405) -> (-2.1687, 1.2333) projected
  line L712 (-2.1687, 1.2333) -> (-2.156, 1.2266) projected
  line L713 (-2.156, 1.2266) -> (-2.1433, 1.2205) projected
  line L714 (-2.1433, 1.2205) -> (-2.1305, 1.2151) projected
  line L715 (-2.1305, 1.2151) -> (-2.1241, 1.2126) projected
  line L716 (-2.1241, 1.2126) -> (-2.1208, 1.2114) projected
  line L717 (-2.1208, 1.2114) -> (-2.1176, 1.2103) projected
  line L718 (-2.1176, 1.2103) -> (-2.122, 1.1538) projected
  line L719 (-2.122, 1.1538) -> (-2.1254, 1.1532) projected
  point P0 (0, 0)
body "Solid1"
